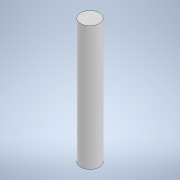
# Autodesk Inventor part: 零件3
Saved by Autodesk Inventor 2022 (Build 260153000, 153)
## iProperties
Created: 2023-03-09
Part Number: 零件3
Material: 一般
Document SubType Name: Modeling
Designer: JOU
Density: 1 g/cm^3
Appearance: 預設
Author: JOU
Autodesk Inventor part; units mm, degrees
ref_plane "YZ Plane" through (0, 0, 0) normal (1, 0, 0) x (0, 1, 0)
ref_plane "XZ Plane" through (0, 0, 0) normal (0, 1, 0) x (-1, 0, 0)
ref_plane "XY Plane" through (0, 0, 0) normal (0, 0, 1) x (1, 0, 0)
sketch "草圖1" plane through (0, 0, 0) normal (0, 1, 0) x (-1, 0, 0)
  circle A0 centre (0.913, -0.7631) radius 0.75
  point P0 (0, 0)
  dimension "d0" = 1.5
  dimension "d0" = 1.5
  constraints: 1 centre point
  measures "d0" diameter of A0
extrude "擠出1" add sketch "草圖1" along normal blind 10
